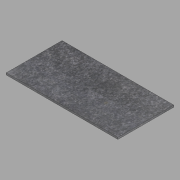
# Autodesk Inventor part: 3 - 1
Saved by Autodesk Inventor 2022.2 (Build 262287000, 287)
## iProperties
Created: 2022-02-24
Part Number: 3 - 1
Material: Granite, Cut, Polished
Document SubType Name: Modeling
Designer: awelt
Mass: 79641.1 g
Surface Area: 24387 cm^2
Volume: 29496.7 cm^3
Density: 2.7 g/cm^3
Appearance: Kasota SN sapphire
Author: awelt
Autodesk Inventor part; units mm, degrees
ref_plane "YZ Plane" through (0, 0, 0) normal (1, 0, 0) x (0, 1, 0)
ref_plane "XZ Plane" through (0, 0, 0) normal (0, 1, 0) x (-1, 0, 0)
ref_plane "XY Plane" through (0, 0, 0) normal (0, 0, 1) x (1, 0, 0)
sketch "Sketch1" plane through (0, 0, 0) normal (0, 1, 0) x (-1, 0, 0)
  line L0 (762, -381) -> (-762, -381)
  line L1 (-762, -381) -> (-762, 381)
  line L2 (-762, 381) -> (762, 381)
  line L3 (762, 381) -> (762, -381)
  line L4 (762, -381) -> (-762, 381) construction
  line L5 (-762, -381) -> (762, 381) construction
  point P0 (0, 0)
  dimension "d0" = 1524
  dimension "d1" = 762
  constraints: 12 end point, 2 midpoint, 2 parallel, 1 horizontal, 1 perpendicular
  measures "d0" distance of L1.end L2.end
  measures "d1" distance of L0.end L1.end
extrude "Extrusion1" add sketch "Sketch1" along normal blind 25.4
body "Solid1"
